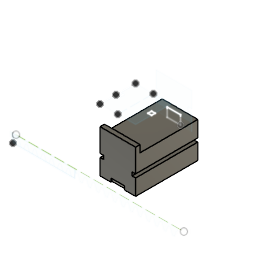
Base Piston_v6 (Autodesk Fusion 360 design; units mm, degrees)
description: Rack Gear; Module: 3.000000; Number of Teeth: 20; Pressure Angle: 20.000000; Root Fillet Radius: 0.040000; Clearance: 0.000000; Gear Thickness: 0.800000; Height: 1.000000;
Autodesk Fusion 360 part; units mm, degrees
sketch "Szkic1" plane through (0, 0, 0) normal (1, 0, 0) x (0, 1, 0)
  line L0 (0, 0) -> (40, 0)
  line L1 (40, 0) -> (40, 70)
  line L2 (40, 70) -> (0, 70)
  line L3 (0, 70) -> (0, 0)
  dimension "d1" = 40
  dimension "d2" = 70
  constraint horizontal L0
  constraint vertical L1
  constraint horizontal L2
  constraint vertical L3
  constraint coincident L0.start L3.end
  measures "d1" distance of L0.start L0.end
  measures "d2" distance of L0.start L2.end
extrude "Wyciągnięcie proste1" add sketch "Szkic1" along normal blind 40 makes body 1
sketch "Szkic2" plane through (0, 0, 70) normal (0, 0, 1) x (-1, 0, 0)
  line L0 (0, -40) -> (0, 0)
  line L1 (0, 0) -> (-40, 0)
  line L2 (-40, 0) -> (-40, -40)
  line L3 (-40, -40) -> (0, -40)
  line L4 (-20, 0) -> (-20, -40) construction
  line L5 (0, -18) -> (-4, -18)
  line L6 (-4, -18) -> (-4, -22)
  line L7 (-4, -22) -> (0, -22)
  line L8 (0, -22) -> (0, -18)
  line L9 (0, -40) -> (0, -22)
  line L10 (0, 0) -> (0, -18)
  line L11 (-36, -22) -> (-40, -22)
  line L12 (-40, -22) -> (-40, -18)
  line L13 (-36, -18) -> (-36, -22)
  line L14 (-40, -18) -> (-36, -18)
  dimension "d5" = 20
  dimension "d6" = 4
  dimension "d7" = 4
  constraint coincident L1 L4.start
  constraint coincident L3 L4.end
  constraint perpendicular L3 L4
  constraint horizontal L5
  constraint vertical L6
  constraint horizontal L7
  constraint vertical L8
  constraint coincident L0 L5.start
  constraint coincident L0.start L3.end
  constraint perpendicular L7 L9
  constraint coincident L0.end L1.start
  constraint perpendicular L1 L10
  constraint equal L9 L10
  constraint symmetric L4 L5.start L12.end
  constraint symmetric L4 L5.end L13.start
  constraint symmetric L4 L6.end L11.start
  constraint symmetric L4 L7.end L11.end
  measures "d5" distance of L0 L4
  measures "d6" distance of L5.start L5.end
  measures "d7" distance of L5.start L7.end
extrude "Wyciągnięcie proste2" cut sketch "Szkic2" against normal through all contours L0 L5 L6 L7 L8 | L2 L11 L12 L13 L14 bodies 1
sketch "Szkic3" plane through (0, 0, 0) normal (0, -1, 0) x (1, 0, 0)
  line L0 (0, 70) -> (0, 0)
  line L1 (0, 0) -> (40, 0)
  line L2 (40, 0) -> (40, 70)
  line L3 (40, 70) -> (0, 70)
  line L4 (0, 0) -> (40, 0)
  line L5 (40, 0) -> (40, 5)
  line L6 (40, 5) -> (0, 5)
  line L7 (0, 5) -> (0, 0)
  constraint horizontal L4
  constraint vertical L5
  constraint horizontal L6
  constraint vertical L7
  constraint coincident L2 L5.end
  constraint coincident L0.end L1.start
extrude "Wyciągnięcie proste3" add sketch "Szkic3" along normal blind 8 contours L0 L1 L2 L4 L5 L6 L7 bodies 1
move_body "Move1" bodies 1 to x (1, 0, 0) y (0, 0, -1) z (0, 1, 0) at (0, -7.0016, 71.7867)
sketch "Sketch4" plane through (0, 62.9984, 0) normal (0, 1, 0) x (-1, 0, 0)
  line L0 (0, 49.7867) -> (-4, 49.7867)
  line L1 (-4, 49.7867) -> (-4, 53.7867)
  line L2 (-4, 53.7867) -> (0, 53.7867)
  line L3 (0, 53.7867) -> (0, 71.7867)
  line L4 (0, 71.7867) -> (-40, 71.7867)
  line L5 (-40, 71.7867) -> (-40, 53.7867)
  line L6 (-40, 53.7867) -> (-36, 53.7867)
  line L7 (-36, 53.7867) -> (-36, 49.7867)
  line L8 (-36, 49.7867) -> (-40, 49.7867)
  line L9 (-40, 49.7867) -> (-40, 31.7867)
  line L10 (-40, 31.7867) -> (0, 31.7867)
  line L11 (0, 31.7867) -> (0, 49.7867)
  line L12 (-27.5, 31.7867) -> (-12.5, 31.7867)
  line L13 (-12.5, 31.7867) -> (-12.5, 41.7867)
  line L14 (-12.5, 41.7867) -> (-27.5, 41.7867)
  line L15 (-27.5, 41.7867) -> (-27.5, 31.7867)
  dimension "d14" = 15
  dimension "d15" = 10
  dimension "d16" = 12.5
  constraint horizontal L12
  constraint vertical L13
  constraint horizontal L14
  constraint vertical L15
  constraint coincident L10 L12.start
  measures "d14" distance of L12.start L12.end
  measures "d15" distance of L12.start L14.end
  measures "d16" distance of L9 L15
extrude "Extrude4" cut sketch "Sketch4" against normal through all contours L10 L12 L13 L14 L15 bodies 1
sketch "Sketch1" plane through (0, 0, 0) normal (0, 1, 0) x (1, 0, 0) in component "Rack Gear (20 teeth)"
  line L0 (-48.211, 3.5132) -> (-50.572, 10)
  arc A0 (-55.4616, 3.5132) -> (-55.8374, 3.25) centre (-55.8374, 3.65) cw
  line L1 (-65.2622, 3.25) -> (-66.6847, 3.25)
  line L2 (-71.9501, 10) -> (-74.3111, 3.5132)
  arc A1 (-46.0368, 3.5132) -> (-46.4127, 3.25) centre (-46.4127, 3.65) cw
  arc A2 (-64.8863, 3.5132) -> (-65.2622, 3.25) centre (-65.2622, 3.65) cw
  arc A3 (-74.3111, 3.5132) -> (-74.687, 3.25) centre (-74.687, 3.65) cw
  arc A4 (93.5366, 3.25) -> (93.1607, 3.5132) centre (93.5366, 3.65) cw
  line L3 (76.1094, 3.25) -> (74.687, 3.25)
  line L4 (90.7997, 10) -> (88.2711, 10)
  arc A5 (85.9101, 3.5132) -> (85.5342, 3.25) centre (85.5342, 3.65) cw
  arc A6 (84.1118, 3.25) -> (83.7359, 3.5132) centre (84.1118, 3.65) cw
  line L5 (5.9767, 10) -> (3.4481, 10)
  arc A7 (-10.136, 3.25) -> (-10.5119, 3.5132) centre (-10.136, 3.65) cw
  line L6 (15.4015, 10) -> (12.8729, 10)
  line L7 (71.9501, 10) -> (69.4215, 10)
  line L8 (94.2478, 3.25) -> (93.5366, 3.25)
  line L9 (85.5342, 3.25) -> (84.1118, 3.25)
  line L10 (-1.0871, 3.5132) -> (-3.4481, 10)
  line L11 (-10.5119, 3.5132) -> (-12.8729, 10)
  line L12 (93.1607, 3.5132) -> (90.7997, 10)
  line L13 (88.2711, 10) -> (85.9101, 3.5132)
  line L14 (83.7359, 3.5132) -> (81.3749, 10)
  line L15 (78.8463, 10) -> (76.4853, 3.5132)
  line L16 (81.3749, 10) -> (78.8463, 10)
  arc A8 (76.4853, 3.5132) -> (76.1094, 3.25) centre (76.1094, 3.65) cw
  arc A9 (74.687, 3.25) -> (74.3111, 3.5132) centre (74.687, 3.65) cw
  line L17 (74.3111, 3.5132) -> (71.9501, 10)
  arc A10 (67.0605, 3.5132) -> (66.6847, 3.25) centre (66.6847, 3.65) cw
  arc A11 (18.1383, 3.25) -> (17.7625, 3.5132) centre (18.1383, 3.65) cw
  line L18 (38.4103, 3.25) -> (36.9879, 3.25)
  arc A12 (65.2622, 3.25) -> (64.8863, 3.5132) centre (65.2622, 3.65) cw
  arc A13 (-28.9856, 3.25) -> (-29.3614, 3.5132) centre (-28.9856, 3.65) cw
  arc A14 (27.5631, 3.25) -> (27.1872, 3.5132) centre (27.5631, 3.65) cw
  line L19 (-24.8262, 10) -> (-27.1872, 3.5132)
  line L20 (0.7112, 3.25) -> (-0.7112, 3.25)
  arc A15 (29.3614, 3.5132) -> (28.9856, 3.25) centre (28.9856, 3.65) cw
  line L21 (69.4215, 10) -> (67.0605, 3.5132)
  line L22 (64.8863, 3.5132) -> (62.5253, 10)
  line L23 (22.2977, 10) -> (19.9367, 3.5132)
  line L24 (41.1472, 10) -> (38.7862, 3.5132)
  arc A16 (57.6358, 3.5132) -> (57.2599, 3.25) centre (57.2599, 3.65) cw
  arc A17 (-27.1872, 3.5132) -> (-27.5631, 3.25) centre (-27.5631, 3.65) cw
  line L25 (53.1006, 10) -> (50.572, 10)
  line L26 (34.251, 10) -> (31.7224, 10)
  line L27 (27.1872, 3.5132) -> (24.8262, 10)
  arc A18 (55.8374, 3.25) -> (55.4616, 3.5132) centre (55.8374, 3.65) cw
  line L28 (-18.1383, 3.25) -> (-19.5608, 3.25)
  line L29 (3.4481, 10) -> (1.0871, 3.5132)
  line L30 (-19.9367, 3.5132) -> (-22.2977, 10)
  arc A19 (-19.5608, 3.25) -> (-19.9367, 3.5132) centre (-19.5608, 3.65) cw
  line L31 (-27.5631, 3.25) -> (-28.9856, 3.25)
  line L32 (-12.8729, 10) -> (-15.4015, 10)
  line L33 (-15.4015, 10) -> (-17.7625, 3.5132)
  arc A20 (10.5119, 3.5132) -> (10.136, 3.25) centre (10.136, 3.65) cw
  arc A21 (46.4127, 3.25) -> (46.0368, 3.5132) centre (46.4127, 3.65) cw
  line L34 (47.8351, 3.25) -> (46.4127, 3.25)
  line L35 (36.612, 3.5132) -> (34.251, 10)
  arc A22 (8.7136, 3.25) -> (8.3377, 3.5132) centre (8.7136, 3.65) cw
  arc A23 (-0.7112, 3.25) -> (-1.0871, 3.5132) centre (-0.7112, 3.65) cw
  arc A24 (-17.7625, 3.5132) -> (-18.1383, 3.25) centre (-18.1383, 3.65) cw
  line L36 (-5.9767, 10) -> (-8.3377, 3.5132)
  arc A25 (19.9367, 3.5132) -> (19.5608, 3.25) centre (19.5608, 3.65) cw
  line L37 (-22.2977, 10) -> (-24.8262, 10)
  line L38 (57.2599, 3.25) -> (55.8374, 3.25)
  line L39 (-74.687, 3.25) -> (-76.1094, 3.25)
  line L40 (-78.8463, 10) -> (-81.3749, 10)
  line L41 (-59.9968, 10) -> (-62.5253, 10)
  arc A26 (-57.2599, 3.25) -> (-57.6358, 3.5132) centre (-57.2599, 3.65) cw
  line L42 (19.5608, 3.25) -> (18.1383, 3.25)
  line L43 (-62.5253, 10) -> (-64.8863, 3.5132)
  line L44 (-81.3749, 10) -> (-83.7359, 3.5132)
  line L45 (-3.4481, 10) -> (-5.9767, 10)
  line L46 (10.136, 3.25) -> (8.7136, 3.25)
  line L47 (62.5253, 10) -> (59.9968, 10)
  line L48 (50.572, 10) -> (48.211, 3.5132)
  arc A27 (48.211, 3.5132) -> (47.8351, 3.25) centre (47.8351, 3.65) cw
  arc A28 (-38.4103, 3.25) -> (-38.7862, 3.5132) centre (-38.4103, 3.65) cw
  arc A29 (-83.7359, 3.5132) -> (-84.1118, 3.25) centre (-84.1118, 3.65) cw
  line L49 (-69.4215, 10) -> (-71.9501, 10)
  line L50 (-67.0605, 3.5132) -> (-69.4215, 10)
  line L51 (31.7224, 10) -> (29.3614, 3.5132)
  line L52 (-38.7862, 3.5132) -> (-41.1472, 10)
  line L53 (28.9856, 3.25) -> (27.5631, 3.25)
  arc A30 (-76.1094, 3.25) -> (-76.4853, 3.5132) centre (-76.1094, 3.65) cw
  line L54 (-93.5366, 3.25) -> (-94.2478, 3.25)
  arc A31 (36.9879, 3.25) -> (36.612, 3.5132) centre (36.9879, 3.65) cw
  line L55 (-76.4853, 3.5132) -> (-78.8463, 10)
  line L56 (-41.1472, 10) -> (-43.6758, 10)
  line L57 (-90.7997, 10) -> (-93.1607, 3.5132)
  line L58 (46.0368, 3.5132) -> (43.6758, 10)
  line L59 (66.6847, 3.25) -> (65.2622, 3.25)
  line L60 (-94.2478, 3.25) -> (-94.2478, 0)
  line L61 (94.2478, 0) -> (94.2478, 3.25)
  line L62 (-8.7136, 3.25) -> (-10.136, 3.25)
  arc A32 (38.7862, 3.5132) -> (38.4103, 3.25) centre (38.4103, 3.65) cw
  line L63 (-31.7224, 10) -> (-34.251, 10)
  line L64 (-55.8374, 3.25) -> (-57.2599, 3.25)
  arc A33 (-85.5342, 3.25) -> (-85.9101, 3.5132) centre (-85.5342, 3.65) cw
  line L65 (17.7625, 3.5132) -> (15.4015, 10)
  line L66 (12.8729, 10) -> (10.5119, 3.5132)
  line L67 (43.6758, 10) -> (41.1472, 10)
  line L68 (-94.2478, 0) -> (94.2478, 0)
  arc A34 (-93.1607, 3.5132) -> (-93.5366, 3.25) centre (-93.5366, 3.65) cw
  line L69 (-50.572, 10) -> (-53.1006, 10)
  line L70 (24.8262, 10) -> (22.2977, 10)
  line L71 (-36.9879, 3.25) -> (-38.4103, 3.25)
  arc A35 (-47.8351, 3.25) -> (-48.211, 3.5132) centre (-47.8351, 3.65) cw
  line L72 (-29.3614, 3.5132) -> (-31.7224, 10)
  arc A36 (-66.6847, 3.25) -> (-67.0605, 3.5132) centre (-66.6847, 3.65) cw
  arc A37 (-8.3377, 3.5132) -> (-8.7136, 3.25) centre (-8.7136, 3.65) cw
  line L73 (59.9968, 10) -> (57.6358, 3.5132)
  line L74 (-43.6758, 10) -> (-46.0368, 3.5132)
  line L75 (-88.2711, 10) -> (-90.7997, 10)
  line L76 (55.4616, 3.5132) -> (53.1006, 10)
  line L77 (-57.6358, 3.5132) -> (-59.9968, 10)
  line L78 (8.3377, 3.5132) -> (5.9767, 10)
  arc A38 (1.0871, 3.5132) -> (0.7112, 3.25) centre (0.7112, 3.65) cw
  line L79 (-34.251, 10) -> (-36.612, 3.5132)
  line L80 (-85.9101, 3.5132) -> (-88.2711, 10)
  line L81 (-46.4127, 3.25) -> (-47.8351, 3.25)
  arc A39 (-36.612, 3.5132) -> (-36.9879, 3.25) centre (-36.9879, 3.65) cw
  line L82 (-53.1006, 10) -> (-55.4616, 3.5132)
  line L83 (-84.1118, 3.25) -> (-85.5342, 3.25)
extrude "Extrude1" add sketch "Sketch1" along normal blind 8 separate body makes body 2 in component "Rack Gear (20 teeth)"
sketch "Sketch2" plane through (0, 0, 0) normal (0, 1, 0) x (1, 0, 0) in component "Rack Gear (20 teeth)"
  line L0 (-94.2578, 7) -> (94.2578, 7) construction
extrude "Extrude2" add 1 faces at (52.2577, 0, -5.6755) along direction (0, -1, 0) blind 7 on bodies 2 bodies 2 in component "Rack Gear (20 teeth)"
sketch "Sketch5" plane through (0, -7, 0) normal (0, -1, 0) x (1, 0, 0)
  line L0 (-85.5342, -3.25) -> (-84.1118, -3.25)
  arc A0 (-83.7359, -3.5132) -> (-84.1118, -3.25) centre (-84.1118, -3.65) ccw
  line L1 (-83.7359, -3.5132) -> (-81.3749, -10)
  line L2 (-81.3749, -10) -> (-78.8463, -10)
  line L3 (-78.8463, -10) -> (-76.4853, -3.5132)
  arc A1 (-76.1094, -3.25) -> (-76.4853, -3.5132) centre (-76.1094, -3.65) ccw
  line L4 (-76.1094, -3.25) -> (-74.687, -3.25)
  arc A2 (-74.3111, -3.5132) -> (-74.687, -3.25) centre (-74.687, -3.65) ccw
  line L5 (-74.3111, -3.5132) -> (-71.9501, -10)
  line L6 (-71.9501, -10) -> (-69.4215, -10)
  line L7 (-69.4215, -10) -> (-67.0605, -3.5132)
  arc A3 (-66.6847, -3.25) -> (-67.0605, -3.5132) centre (-66.6847, -3.65) ccw
  line L8 (-66.6847, -3.25) -> (-65.2622, -3.25)
  arc A4 (-64.8863, -3.5132) -> (-65.2622, -3.25) centre (-65.2622, -3.65) ccw
  line L9 (-64.8863, -3.5132) -> (-62.5253, -10)
  line L10 (-62.5253, -10) -> (-59.9968, -10)
  line L11 (-59.9968, -10) -> (-57.6358, -3.5132)
  arc A5 (-57.2599, -3.25) -> (-57.6358, -3.5132) centre (-57.2599, -3.65) ccw
  line L12 (-57.2599, -3.25) -> (-55.8374, -3.25)
  arc A6 (-55.4616, -3.5132) -> (-55.8374, -3.25) centre (-55.8374, -3.65) ccw
  line L13 (-55.4616, -3.5132) -> (-53.1006, -10)
  line L14 (-53.1006, -10) -> (-50.572, -10)
  line L15 (-50.572, -10) -> (-48.211, -3.5132)
  arc A7 (-47.8351, -3.25) -> (-48.211, -3.5132) centre (-47.8351, -3.65) ccw
  line L16 (-47.8351, -3.25) -> (-46.4127, -3.25)
  arc A8 (-46.0368, -3.5132) -> (-46.4127, -3.25) centre (-46.4127, -3.65) ccw
  line L17 (-46.0368, -3.5132) -> (-43.6758, -10)
  line L18 (-43.6758, -10) -> (-41.1472, -10)
  line L19 (-41.1472, -10) -> (-38.7862, -3.5132)
  arc A9 (-38.4103, -3.25) -> (-38.7862, -3.5132) centre (-38.4103, -3.65) ccw
  line L20 (-38.4103, -3.25) -> (-36.9879, -3.25)
  arc A10 (-36.612, -3.5132) -> (-36.9879, -3.25) centre (-36.9879, -3.65) ccw
  line L21 (-36.612, -3.5132) -> (-34.251, -10)
  line L22 (-34.251, -10) -> (-31.7224, -10)
  line L23 (-31.7224, -10) -> (-29.3614, -3.5132)
  arc A11 (-28.9856, -3.25) -> (-29.3614, -3.5132) centre (-28.9856, -3.65) ccw
  line L24 (-28.9856, -3.25) -> (-27.5631, -3.25)
  arc A12 (-27.1872, -3.5132) -> (-27.5631, -3.25) centre (-27.5631, -3.65) ccw
  line L25 (-27.1872, -3.5132) -> (-24.8262, -10)
  line L26 (-24.8262, -10) -> (-22.2977, -10)
  line L27 (-22.2977, -10) -> (-19.9367, -3.5132)
  arc A13 (-19.5608, -3.25) -> (-19.9367, -3.5132) centre (-19.5608, -3.65) ccw
  line L28 (-19.5608, -3.25) -> (-18.1383, -3.25)
  arc A14 (-17.7625, -3.5132) -> (-18.1383, -3.25) centre (-18.1383, -3.65) ccw
  line L29 (-17.7625, -3.5132) -> (-15.4015, -10)
  line L30 (-15.4015, -10) -> (-12.8729, -10)
  line L31 (-12.8729, -10) -> (-10.5119, -3.5132)
  arc A15 (-10.136, -3.25) -> (-10.5119, -3.5132) centre (-10.136, -3.65) ccw
  line L32 (-10.136, -3.25) -> (-8.7136, -3.25)
  arc A16 (-8.3377, -3.5132) -> (-8.7136, -3.25) centre (-8.7136, -3.65) ccw
  line L33 (-8.3377, -3.5132) -> (-5.9767, -10)
  line L34 (-5.9767, -10) -> (-3.4481, -10)
  line L35 (-3.4481, -10) -> (-1.0871, -3.5132)
  arc A17 (-0.7112, -3.25) -> (-1.0871, -3.5132) centre (-0.7112, -3.65) ccw
  line L36 (-0.7112, -3.25) -> (0.7112, -3.25)
  arc A18 (1.0871, -3.5132) -> (0.7112, -3.25) centre (0.7112, -3.65) ccw
  line L37 (1.0871, -3.5132) -> (3.4481, -10)
  line L38 (3.4481, -10) -> (5.9767, -10)
  line L39 (5.9767, -10) -> (8.3377, -3.5132)
  arc A19 (8.7136, -3.25) -> (8.3377, -3.5132) centre (8.7136, -3.65) ccw
  line L40 (8.7136, -3.25) -> (10.136, -3.25)
  arc A20 (10.5119, -3.5132) -> (10.136, -3.25) centre (10.136, -3.65) ccw
  line L41 (10.5119, -3.5132) -> (12.8729, -10)
  line L42 (12.8729, -10) -> (15.4015, -10)
  line L43 (15.4015, -10) -> (17.7625, -3.5132)
  arc A21 (18.1383, -3.25) -> (17.7625, -3.5132) centre (18.1383, -3.65) ccw
  line L44 (18.1383, -3.25) -> (19.5608, -3.25)
  arc A22 (19.9367, -3.5132) -> (19.5608, -3.25) centre (19.5608, -3.65) ccw
  line L45 (19.9367, -3.5132) -> (22.2977, -10)
  line L46 (22.2977, -10) -> (24.8262, -10)
  line L47 (24.8262, -10) -> (27.1872, -3.5132)
  arc A23 (27.5631, -3.25) -> (27.1872, -3.5132) centre (27.5631, -3.65) ccw
  line L48 (27.5631, -3.25) -> (28.9856, -3.25)
  arc A24 (29.3614, -3.5132) -> (28.9856, -3.25) centre (28.9856, -3.65) ccw
  line L49 (29.3614, -3.5132) -> (31.7224, -10)
  line L50 (31.7224, -10) -> (34.251, -10)
  line L51 (34.251, -10) -> (36.612, -3.5132)
  arc A25 (36.9879, -3.25) -> (36.612, -3.5132) centre (36.9879, -3.65) ccw
  line L52 (36.9879, -3.25) -> (38.4103, -3.25)
  arc A26 (38.7862, -3.5132) -> (38.4103, -3.25) centre (38.4103, -3.65) ccw
  line L53 (38.7862, -3.5132) -> (41.1472, -10)
  line L54 (41.1472, -10) -> (43.6758, -10)
  line L55 (43.6758, -10) -> (46.0368, -3.5132)
  arc A27 (46.4127, -3.25) -> (46.0368, -3.5132) centre (46.4127, -3.65) ccw
  line L56 (46.4127, -3.25) -> (47.8351, -3.25)
  arc A28 (48.211, -3.5132) -> (47.8351, -3.25) centre (47.8351, -3.65) ccw
  line L57 (48.211, -3.5132) -> (50.572, -10)
  line L58 (50.572, -10) -> (53.1006, -10)
  line L59 (53.1006, -10) -> (55.4616, -3.5132)
  arc A29 (55.8374, -3.25) -> (55.4616, -3.5132) centre (55.8374, -3.65) ccw
  line L60 (55.8374, -3.25) -> (57.2599, -3.25)
  arc A30 (57.6358, -3.5132) -> (57.2599, -3.25) centre (57.2599, -3.65) ccw
  line L61 (57.6358, -3.5132) -> (59.9968, -10)
  line L62 (59.9968, -10) -> (62.5253, -10)
  line L63 (62.5253, -10) -> (64.8863, -3.5132)
  arc A31 (65.2622, -3.25) -> (64.8863, -3.5132) centre (65.2622, -3.65) ccw
  line L64 (65.2622, -3.25) -> (66.6847, -3.25)
  arc A32 (67.0605, -3.5132) -> (66.6847, -3.25) centre (66.6847, -3.65) ccw
  line L65 (67.0605, -3.5132) -> (69.4215, -10)
  line L66 (69.4215, -10) -> (71.9501, -10)
  line L67 (71.9501, -10) -> (74.3111, -3.5132)
  arc A33 (74.687, -3.25) -> (74.3111, -3.5132) centre (74.687, -3.65) ccw
  line L68 (74.687, -3.25) -> (76.1094, -3.25)
  arc A34 (76.4853, -3.5132) -> (76.1094, -3.25) centre (76.1094, -3.65) ccw
  line L69 (76.4853, -3.5132) -> (78.8463, -10)
  line L70 (78.8463, -10) -> (81.3749, -10)
  line L71 (81.3749, -10) -> (83.7359, -3.5132)
  arc A35 (84.1118, -3.25) -> (83.7359, -3.5132) centre (84.1118, -3.65) ccw
  line L72 (84.1118, -3.25) -> (85.5342, -3.25)
  arc A36 (85.9101, -3.5132) -> (85.5342, -3.25) centre (85.5342, -3.65) ccw
  line L73 (85.9101, -3.5132) -> (88.2711, -10)
  line L74 (88.2711, -10) -> (90.7997, -10)
  line L75 (90.7997, -10) -> (93.1607, -3.5132)
  arc A37 (93.5366, -3.25) -> (93.1607, -3.5132) centre (93.5366, -3.65) ccw
  line L76 (93.5366, -3.25) -> (94.2478, -3.25)
  line L77 (94.2478, -3.25) -> (94.2478, 0)
  line L78 (94.2478, 0) -> (-94.2478, 0)
  line L79 (-94.2478, 0) -> (-94.2478, -3.25)
  line L80 (-94.2478, -3.25) -> (-93.5366, -3.25)
  arc A38 (-93.1607, -3.5132) -> (-93.5366, -3.25) centre (-93.5366, -3.65) ccw
  line L81 (-93.1607, -3.5132) -> (-90.7997, -10)
  line L82 (-90.7997, -10) -> (-88.2711, -10)
  line L83 (-88.2711, -10) -> (-85.9101, -3.5132)
  arc A39 (-85.5342, -3.25) -> (-85.9101, -3.5132) centre (-85.5342, -3.65) ccw
  line L84 (-90.7997, -10) -> (-20.7997, -10)
  line L85 (-20.7997, -10) -> (-20.7997, 0)
  line L86 (-20.7997, 0) -> (-90.7997, 0)
  line L87 (-90.7997, 0) -> (-90.7997, -10)
  dimension "d22" = 70
  dimension "d23" = 10
  constraint horizontal L84
  constraint vertical L85
  constraint horizontal L86
  constraint vertical L87
  constraint coincident L81.end L82.start
  measures "d22" distance of L81.end L84.end
  measures "d23" distance of L81.end L86.end
extrude "Extrude3" cut sketch "Sketch5" against normal blind 24 contours L0 A0 L1 L2 L3 A1 L4 A2 L5 L6 L7 A3 L8 A4 L9 L10 L11 A5 L12 A6 L13 L14 L15 A7 L16 A8 L17 L18 L19 A9 L20 A10 L21 L22 L23 A11 L24 A12 L25 L26 L27 L78 L82 L83 A39 L84 L85 L86 L87 keep common part bodies 2 in component "Rack Gear (20 teeth)"
move_body "Move3" bodies 1 to x (1, 0, 0) y (0, 1, 0) z (0, 0, 1) at (0, 7.0016, -31.7867)
move_body "Move3'" bodies 2 to x (1, 0, 0) y (0, 1, 0) z (0, 0, 1) at (118.2997, 62, 10) in component "Rack Gear (20 teeth)"
move_body "Move4" bodies 2 to x (0, -1, 0) y (1, 0, 0) z (0, 0, 1) at (-42.5, 97.5, 0) in component "Rack Gear (20 teeth)"
combine "Combine1" operation add target body 1 tool bodies 2
ref_plane "WorkPlane1" through (20, 67, 20) normal (0, 1, 0) x (0, 0, 1)
sketch "Sketch6" plane through (0, 67, 0) normal (0, 1, 0) x (1, 0, 0)
  line L0 (40, 0) -> (0, 0)
  line L1 (0, 0) -> (0, -18)
  line L2 (0, -18) -> (4, -18)
  line L3 (4, -18) -> (4, -22)
  line L4 (4, -22) -> (0, -22)
  line L5 (0, -22) -> (0, -40)
  line L6 (0, -40) -> (40, -40)
  line L7 (40, -40) -> (40, -22)
  line L8 (40, -22) -> (36, -22)
  line L9 (36, -22) -> (36, -18)
  line L10 (36, -18) -> (40, -18)
  line L11 (40, -18) -> (40, 0)
  line L12 (7, -29.4944) -> (7, -10)
  line L13 (7, -10) -> (33, -10)
  line L14 (33, -10) -> (33, -29.4944)
  line L15 (33, -29.4944) -> (20, -37)
  line L16 (20, -37) -> (20, -39) construction
  line L17 (7, -29.4944) -> (20, -37)
  dimension "d31" = 10
  dimension "d32" = 3
  dimension "d33" = 3
  dimension "d36" = 3
  dimension "d37" = 15.0111
  constraint vertical L12
  constraint horizontal L13
  constraint vertical L14
  constraint symmetric L14.end L16 L12.start
  constraint symmetric L15.end L16 L17.end
  measures "d31" distance of L0 L13
  measures "d32" distance of L3 L12
  measures "d33" distance of L9 L14
  measures "d36" distance of L6 L15.end
  measures "d37" distance of L14.end L15.end
extrude "Extrude5" [suppressed]
fillet "Fillet1" [suppressed]
sketch "Sketch7" plane through (0, 0, 40) normal (0, 0, 1) x (-1, 0, 0)
  line L0 (-39.5, -5) -> (-39.5, -69.0001)
  arc A0 (-39.5, -69.0001) -> (-39.0001, -69.5) centre (-39.0001, -69.0001) ccw
  line L1 (-39.0001, -69.5) -> (-0.9999, -69.5)
  arc A1 (-0.9999, -69.5) -> (-0.5, -69.0001) centre (-0.9999, -69.0001) ccw
  line L2 (-0.5, -69.0001) -> (-0.5, -5)
  line L3 (-0.5, -5) -> (-39.5, -5)
  line L4 (-5, -17) -> (-35, -17) construction
  line L5 (-35, -17) -> (-35, -30) construction
  line L6 (-35, -30) -> (-5, -30) construction
  line L7 (-5, -30) -> (-5, -17) construction
  dimension "d42" = 7
extrude "Extrude6" [suppressed]
fillet "Fillet2" [suppressed]
sketch "Sketch8" plane through (0, 0, 0) normal (0, 0, -1) x (1, 0, 0)
  line L0 (28, -3.6765) -> (28, -11.2729)
  line L1 (28, -11.2729) -> (12, -11.2729)
  line L2 (12, -11.2729) -> (12, -3.6765)
  line L3 (12, -3.6765) -> (28, -3.6765)
  line L4 (28, -22.526) -> (28, -30.1224)
  line L5 (28, -30.1224) -> (12, -30.1224)
  line L6 (12, -30.1224) -> (12, -22.526)
  line L7 (12, -22.526) -> (28, -22.526)
  line L8 (28, -41.3756) -> (28, -48.972)
  line L9 (28, -48.972) -> (12, -48.972)
  line L10 (12, -48.972) -> (12, -41.3756)
  line L11 (12, -41.3756) -> (28, -41.3756)
  line L12 (12, -67.8215) -> (12, -60.2251)
  line L13 (12, -60.2251) -> (28, -60.2251)
  line L14 (28, -60.2251) -> (28, -67.8215)
  line L15 (28, -67.8215) -> (12, -67.8215)
  line L16 (28, -50.8003) -> (28, -58.3968)
  line L17 (28, -58.3968) -> (12, -58.3968)
  line L18 (12, -58.3968) -> (12, -50.8003)
  line L19 (12, -50.8003) -> (28, -50.8003)
  line L20 (28, -31.9508) -> (28, -39.5472)
  line L21 (28, -39.5472) -> (12, -39.5472)
  line L22 (12, -39.5472) -> (12, -31.9508)
  line L23 (12, -31.9508) -> (28, -31.9508)
  line L24 (28, -13.1012) -> (28, -20.6976)
  line L25 (28, -20.6976) -> (12, -20.6976)
  line L26 (12, -20.6976) -> (12, -13.1012)
  line L27 (12, -13.1012) -> (28, -13.1012)
  arc A0 (12, -0.9999) -> (11.5001, -0.5) centre (11.5001, -0.9999) ccw
  line L28 (11.5001, -0.5) -> (0.9999, -0.5)
  arc A1 (0.9999, -0.5) -> (0.5, -0.9999) centre (0.9999, -0.9999) ccw
  line L29 (0.5, -0.9999) -> (0.5, -69.0001)
  arc A2 (0.5, -69.0001) -> (0.9999, -69.5) centre (0.9999, -69.0001) ccw
  line L30 (0.9999, -69.5) -> (39.0001, -69.5)
  arc A3 (39.0001, -69.5) -> (39.5, -69.0001) centre (39.0001, -69.0001) ccw
  line L31 (39.5, -69.0001) -> (39.5, -0.9999)
  arc A4 (39.5, -0.9999) -> (39.0001, -0.5) centre (39.0001, -0.9999) ccw
  line L32 (39.0001, -0.5) -> (28.4999, -0.5)
  arc A5 (28.4999, -0.5) -> (28, -0.9999) centre (28.4999, -0.9999) ccw
  line L33 (28, -0.9999) -> (28, -1.8481)
  line L34 (28, -1.8481) -> (12, -1.8481)
  line L35 (12, -1.8481) -> (12, -0.9999)
  line L36 (24, -8) -> (24, -16) construction
  line L37 (24, -16) -> (44, -16) construction
  line L38 (44, -16) -> (44, -8) construction
  line L39 (44, -8) -> (24, -8) construction
  dimension "d48" = 3
extrude "Extrude7" [suppressed]
ref_plane "WorkPlane3" through (20, 69, 20) normal (0, 1, 0) x (0, 0, 1)
sketch "Sketch10" plane through (0, 69, 0) normal (0, 1, 0) x (1, 0, 0)
  line L0 (0.9999, -40) -> (39.0001, -40)
  line L1 (39.0001, 0) -> (0.9999, 0)
  line L2 (36, -18) -> (39.0001, -18)
  line L3 (36, -22) -> (36, -18)
  line L4 (39.0001, -22) -> (36, -22)
  line L5 (20, -40) -> (20, 0) construction
  line L6 (39.2, -18.3) -> (36.3, -18.3)
  line L7 (36.3, -18.3) -> (36.3, -21.7)
  line L8 (36.3, -21.7) -> (39.2, -21.7)
  line L9 (39.2, -21.7) -> (39.2, -18.3)
  line L10 (4, -18) -> (0.9999, -18)
  line L11 (3.7, -18.3) -> (3.7, -21.7)
  line L12 (0.9999, -22) -> (4, -22)
  line L13 (4, -22) -> (4, -18)
  line L14 (3.7, -21.7) -> (0.8, -21.7)
  line L15 (0.8, -18.3) -> (3.7, -18.3)
  line L16 (0.8, -21.7) -> (0.8, -18.3)
  dimension "d55" = 0.3
  dimension "d56" = 0.3
  dimension "d57" = 0.3
  constraint midpoint L0 L5.start
  constraint midpoint L1 L5.end
  constraint horizontal L6
  constraint vertical L7
  constraint horizontal L8
  constraint vertical L9
  constraint symmetric L2.start L5 L10.start
  constraint symmetric L2.end L5 L10.end
  constraint symmetric L3.start L5 L12.end
  constraint symmetric L4.start L5 L12.start
  constraint symmetric L5 L6.start L15.start
  constraint symmetric L5 L6.end L11.start
  constraint symmetric L5 L7.end L11.end
  constraint symmetric L5 L8.end L14.end
  measures "d55" distance of L4 L8
  measures "d56" distance of L2 L6
  measures "d57" distance of L3 L7
extrude "Extrude1'" [suppressed] in component "Supports"
pattern_linear "R-Pattern1" [suppressed] in component "Supports"
component "Rack Gear (20 teeth)" placed x (1, 0, 0) y (0, 1, 0) z (0, 0, 1) at (0, 0, 0)
